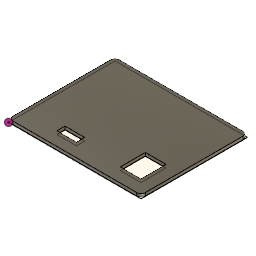
BlimpEnclosureHatchLeonardo v2 (Autodesk Fusion 360 design; units mm, degrees)
Autodesk Fusion 360 part; units mm, degrees
sketch "Sketch1" plane through (0, 0, 0) normal (0, 0, 1) x (1, 0, 0)
  line L0 (0, 0) -> (61, 0)
  line L1 (61, 0) -> (61, 49)
  line L2 (61, 49) -> (0, 49)
  line L3 (0, 49) -> (0, 0)
  line L4 (16, 10) -> (25, 10)
  line L5 (25, 10) -> (25, 6.3)
  line L6 (25, 6.3) -> (16, 6.3)
  line L7 (16, 6.3) -> (16, 10)
  line L8 (45, 18) -> (54.5, 18)
  line L9 (54.5, 18) -> (54.5, 6.5)
  line L10 (54.5, 6.5) -> (45, 6.5)
  line L11 (45, 6.5) -> (45, 18)
  dimension "d1" = 61
  dimension "d2" = 49
  dimension "d3" = 9
  dimension "d4" = 3.7
  dimension "d5" = 10
  dimension "d6" = 16
  dimension "d7" = 9.5
  dimension "d8" = 11.5
  dimension "d9" = 45
  dimension "d10" = 18
  constraint horizontal L0
  constraint vertical L1
  constraint horizontal L2
  constraint vertical L3
  constraint coincident L0.start L3.end
  constraint horizontal L4
  constraint vertical L5
  constraint horizontal L6
  constraint vertical L7
  constraint horizontal L8
  constraint vertical L9
  constraint horizontal L10
  constraint vertical L11
  measures "d1" distance of L0.start L0.end
  measures "d2" distance of L0.start L2.end
  measures "d3" distance of L4.start L4.end
  measures "d4" distance of L4.start L6.end
  measures "d5" distance of L0 L4.start
  measures "d6" distance of L3 L4.start
  measures "d7" distance of L8.start L8.end
  measures "d8" distance of L8.start L10.end
  measures "d9" distance of L3 L8.start
  measures "d10" distance of L0 L8.start
extrude "Extrude1" add sketch "Sketch1" along normal blind 1.5
fillet "Fillet1" radius 2 4 edges at (0, 0, 0.75) (61, 0, 0.75) (61, 49, 0.75) (0, 49, 0.75)
